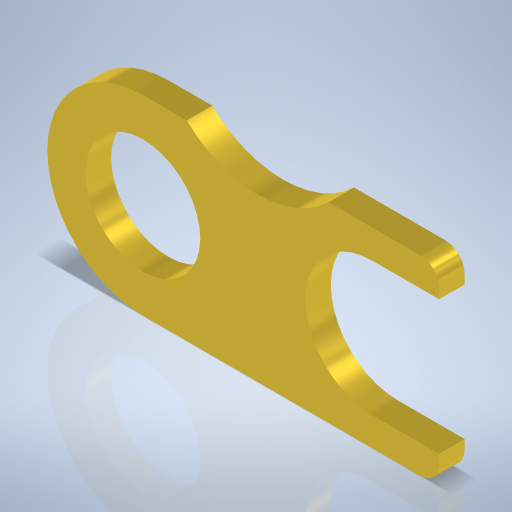
# Autodesk Inventor part: 205 part 3
Saved by Autodesk Inventor 2024 (Build 280153000, 153)
## iProperties
Created: 2024-07-12
Part Number: 205 part 3
Material: Gold
Document SubType Name: Modeling
Designer: ffogue
Density: 19.3 g/cm^3
Appearance: Metall - 2400F (heiß)
Author: ffogue
Autodesk Inventor part; units mm, degrees
ref_plane "YZ Plane" through (0, 0, 0) normal (1, 0, 0) x (0, 1, 0)
ref_plane "XZ Plane" through (0, 0, 0) normal (0, 1, 0) x (-1, 0, 0)
ref_plane "XY Plane" through (0, 0, 0) normal (0, 0, 1) x (1, 0, 0)
sketch "Skizze1" plane through (0, 0, 0) normal (0, 1, 0) x (-1, 0, 0)
  arc A0 (0, -7.5) -> (0, 7.5) centre (0, 0) ccw
  arc A1 (-18, -5.25) -> (-18, 5.25) centre (-18, 0) ccw
  line L0 (0, 7.5) -> (0, -7.5) construction
  line L1 (-18, 5.25) -> (-18, -5.25) construction
  line L2 (-18, 5.25) -> (-23.25, 5.25)
  line L3 (-18, -5.25) -> (-23.25, -5.25)
  line L4 (-23.25, 5.25) -> (-23.25, 6)
  line L5 (-23.25, -5.25) -> (-23.25, -6)
  line L6 (-21.75, -7.5) -> (0, -7.5)
  arc A2 (-21.75, 7.5) -> (-23.25, 6) centre (-21.75, 6) ccw
  arc A3 (-23.25, -6) -> (-21.75, -7.5) centre (-21.75, -6) ccw
  circle A4 centre (-18, 0) radius 5.25 construction
  circle A5 centre (0, 0) radius 4.5
  arc A6 (-14.5621, 7.5) -> (-3.4379, 7.5) centre (-9, 13.25) ccw
  line L7 (-21.75, 7.5) -> (-14.5621, 7.5)
  line L8 (-3.4379, 7.5) -> (0, 7.5)
  point P0 (-23.25, 0)
  point P1 (-9, 5.25)
  dimension "d4" = 10.5
  dimension "d0" = 15
  dimension "d1" = 10.5
  dimension "d2" = 18
  dimension "d3" = 1.5
  dimension "d5" = 9
  dimension "d8" = 8
  dimension "d9" = 9
  constraints: 18 end point, 11 point on circle, 6 centre point, 6 tangent, 3 coincident, 3 horizontal alignment, 3 midpoint, 3 perpendicular, 3 vertical, 3 vertical alignment, 2 horizontal, 1 equal radius, 2 other
  measures "d0" diameter of A0
  measures "d1" diameter of A1
  measures "d2" distance of A1.centre point (0, 0)
  measures "d3" radius of A2
  measures "d5" diameter of A5
  measures "d8" radius of A6
  measures "d9" horizontal distance of A6.centre point (0, 0)
extrude "Extrusion1" add sketch "Skizze1" along normal mid plane 2
